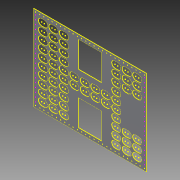
# Autodesk Inventor part: baseplate
Saved by Autodesk Inventor 2014 SP1 (Build 180222100, 222)
## iProperties
Created: 2014-01-05
Part Number: baseplate
Material: Aluminum 6061
Document SubType Name: Sheet Metal
Designer: Arpan
Density: 2.71 g/cm^3
Sheet Metal Rule: Default
Appearance: Aluminum - Flat
Mass: 756.352 g
Surface Area: 3765.33 cm^2
Volume: 279.097 cm^3
Author: Arpan
Autodesk Inventor part; units mm, degrees
ref_plane "YZ Plane" through (0, 0, 0) normal (1, 0, 0) x (0, 1, 0)
ref_plane "XZ Plane" through (0, 0, 0) normal (0, 1, 0) x (-1, 0, 0)
ref_plane "XY Plane" through (0, 0, 0) normal (0, 0, 1) x (1, 0, 0)
sketch "Sketch1" plane through (0, 0, 0) normal (0, 0, 1) x (1, 0, 0)
  line L0 (0, 0) -> (-685.8, 0)
  line L1 (-685.8, 0) -> (-685.8, 516.255)
  line L2 (-685.8, 516.255) -> (0, 516.255)
  line L3 (0, 516.255) -> (0, 0)
  dimension "d0" = 685.8
  dimension "d1" = 516.255
  measures "d0" distance of L1.end L2.end
  measures "d1" distance of L2.end L0.start
extrude "Plate1" add sketch "Sketch1" along normal blind 1.5875
sketch "Sketch4" plane through (0, 0, 1.5875) normal (0, 0, 1) x (1, 0, 0)
  circle A0 centre (-673.1, 503.555) radius 2.0828 projected
  circle A1 centre (-673.1, 12.7) radius 2.0828 projected
extrude "Cut3" cut sketch "Sketch4" against normal blind 1.5875
pattern_linear "Rectangular Pattern2" count 27 spacing 25.4 along (1, 0, 0) of "Cut3"
sketch "Sketch5" plane through (0, 0, 1.5875) normal (0, 0, 1) x (1, 0, 0)
  line L0 (-685.8, 516.255) -> (0, 516.255)
  line L1 (0, 516.255) -> (0, 0)
  line L2 (0, 0) -> (-685.8, 0)
  line L3 (-685.8, 0) -> (-685.8, 516.255)
  line L4 (-25.4, 490.855) -> (-660.4, 490.855)
  line L5 (-660.4, 490.855) -> (-660.4, 25.4)
  line L6 (-660.4, 25.4) -> (-25.4, 25.4)
  line L7 (-25.4, 25.4) -> (-25.4, 490.855)
  line L8 (-660.4, 490.855) -> (-596.9, 490.855)
  line L9 (-596.9, 490.855) -> (-596.9, 444.3095)
  line L10 (-596.9, 444.3095) -> (-660.4, 444.3095)
  line L11 (-660.4, 467.5822) -> (-596.9, 467.5822) construction
  line L12 (-637.1273, 444.3095) -> (-620.1728, 444.3095)
  line L13 (-620.1728, 490.855) -> (-637.1273, 490.855)
  arc A0 (-637.1273, 490.855) -> (-637.1273, 444.3095) centre (-637.1273, 467.5822) ccw
  arc A1 (-620.1728, 444.3095) -> (-620.1728, 490.855) centre (-620.1728, 467.5822) ccw
  line L14 (-620.1728, 487.68) -> (-637.1273, 487.68)
  arc A2 (-637.1273, 487.68) -> (-637.1273, 447.4845) centre (-637.1273, 467.5822) ccw
  line L15 (-637.1273, 447.4845) -> (-620.1728, 447.4845)
  arc A3 (-620.1728, 447.4845) -> (-620.1728, 487.68) centre (-620.1728, 467.5822) ccw
  point P0 (-412.75, 516.255)
  point P1 (-412.75, 0)
  point P2 (-273.05, 0)
  point P3 (-273.05, 516.255)
  point P4 (-628.65, 467.5822)
  dimension "d22" = 25.4
  dimension "d25" = 46.5455
  dimension "d28" = 3.175
  constraints: 34 end point, 10 point on circle, 6 parallel, 5 point on line, 4 centre point, 4 perpendicular, 4 tangent, 2 midpoint, 1 horizontal, 6 other
  measures "d22" distance between parallel lines of L0 L4
  measures "d25" distance of L8.end L9.end
  measures "d28" distance between parallel lines of L8 L14
extrude "Cut5" cut sketch "Sketch5" against normal blind 1.5875 contours A3 L15 A2 L14
pattern_linear "Rectangular Pattern3" count 10 spacing 46.5455 along (0, -1, 0) count 10 spacing 63.5 along (1, 0, 0) of "Cut5"
sketch "Sketch7" plane through (0, 0, 0) normal (0, 0, -1) x (-1, 0, 0)
  line L0 (256.1273, 75.1205) -> (239.1728, 75.1205)
  line L1 (402.7899, 184.15) -> (410.0101, 184.15)
  arc A0 (446.6273, 168.2115) -> (446.6273, 208.407) centre (446.6273, 188.3092) ccw
  arc A1 (429.6728, 208.407) -> (429.6728, 168.2115) centre (429.6728, 188.3092) ccw
  line L2 (412.75, 177.4677) -> (412.75, 152.6053)
  line L3 (273.05, 338.7873) -> (273.05, 363.6497)
  line L4 (283.0101, 332.105) -> (275.7899, 332.105)
  arc A2 (256.1273, 307.848) -> (256.1273, 348.0435) centre (256.1273, 327.9457) ccw
  arc A3 (239.1728, 348.0435) -> (239.1728, 307.848) centre (239.1728, 327.9457) ccw
  line L5 (429.6728, 188.3092) -> (446.6273, 188.3092) construction
  line L6 (429.6728, 168.2115) -> (446.6273, 168.2115)
  line L7 (446.6273, 208.407) -> (429.6728, 208.407)
  arc A4 (429.6728, 208.407) -> (429.6728, 168.2115) centre (429.6728, 188.3092) ccw
  arc A5 (446.6273, 168.2115) -> (446.6273, 208.407) centre (446.6273, 188.3092) ccw
  line L8 (366.1728, 168.2115) -> (383.1273, 168.2115)
  line L9 (383.1273, 208.407) -> (366.1728, 208.407)
  arc A6 (366.1728, 208.407) -> (366.1728, 168.2115) centre (366.1728, 188.3092) ccw
  arc A7 (383.1273, 168.2115) -> (383.1273, 208.407) centre (383.1273, 188.3092) ccw
  line L10 (302.6728, 168.2115) -> (319.6273, 168.2115)
  line L11 (319.6273, 208.407) -> (302.6728, 208.407)
  arc A8 (302.6728, 208.407) -> (302.6728, 168.2115) centre (302.6728, 188.3092) ccw
  arc A9 (319.6273, 168.2115) -> (319.6273, 208.407) centre (319.6273, 188.3092) ccw
  line L12 (239.1728, 168.2115) -> (256.1273, 168.2115)
  line L13 (256.1273, 208.407) -> (239.1728, 208.407)
  arc A10 (239.1728, 208.407) -> (239.1728, 168.2115) centre (239.1728, 188.3092) ccw
  arc A11 (256.1273, 168.2115) -> (256.1273, 208.407) centre (256.1273, 188.3092) ccw
  line L14 (429.6728, 121.666) -> (446.6273, 121.666)
  line L15 (446.6273, 161.8615) -> (429.6728, 161.8615)
  arc A12 (429.6728, 161.8615) -> (429.6728, 121.666) centre (429.6728, 141.7637) ccw
  arc A13 (446.6273, 121.666) -> (446.6273, 161.8615) centre (446.6273, 141.7637) ccw
  line L16 (366.1728, 121.666) -> (383.1273, 121.666)
  line L17 (383.1273, 161.8615) -> (366.1728, 161.8615)
  arc A14 (366.1728, 161.8615) -> (366.1728, 121.666) centre (366.1728, 141.7637) ccw
  arc A15 (383.1273, 121.666) -> (383.1273, 161.8615) centre (383.1273, 141.7637) ccw
  line L18 (302.6728, 121.666) -> (319.6273, 121.666)
  line L19 (319.6273, 161.8615) -> (302.6728, 161.8615)
  arc A16 (302.6728, 161.8615) -> (302.6728, 121.666) centre (302.6728, 141.7637) ccw
  arc A17 (319.6273, 121.666) -> (319.6273, 161.8615) centre (319.6273, 141.7637) ccw
  line L20 (239.1728, 121.666) -> (256.1273, 121.666)
  line L21 (256.1273, 161.8615) -> (239.1728, 161.8615)
  arc A18 (239.1728, 161.8615) -> (239.1728, 121.666) centre (239.1728, 141.7637) ccw
  arc A19 (256.1273, 121.666) -> (256.1273, 161.8615) centre (256.1273, 141.7637) ccw
  line L22 (429.6728, 75.1205) -> (446.6273, 75.1205)
  line L23 (446.6273, 115.316) -> (429.6728, 115.316)
  arc A20 (429.6728, 115.316) -> (429.6728, 75.1205) centre (429.6728, 95.2182) ccw
  arc A21 (446.6273, 75.1205) -> (446.6273, 115.316) centre (446.6273, 95.2182) ccw
  line L24 (366.1728, 75.1205) -> (383.1273, 75.1205)
  line L25 (383.1273, 115.316) -> (366.1728, 115.316)
  arc A22 (366.1728, 115.316) -> (366.1728, 75.1205) centre (366.1728, 95.2182) ccw
  arc A23 (383.1273, 75.1205) -> (383.1273, 115.316) centre (383.1273, 95.2182) ccw
  line L26 (302.6728, 75.1205) -> (319.6273, 75.1205)
  line L27 (319.6273, 115.316) -> (302.6728, 115.316)
  arc A24 (302.6728, 115.316) -> (302.6728, 75.1205) centre (302.6728, 95.2182) ccw
  arc A25 (319.6273, 75.1205) -> (319.6273, 115.316) centre (319.6273, 95.2182) ccw
  line L28 (239.1728, 75.1205) -> (256.1273, 75.1205)
  line L29 (256.1273, 115.316) -> (239.1728, 115.316)
  arc A26 (239.1728, 115.316) -> (239.1728, 75.1205) centre (239.1728, 95.2182) ccw
  arc A27 (256.1273, 75.1205) -> (256.1273, 115.316) centre (256.1273, 95.2182) ccw
  line L30 (429.6728, 28.575) -> (446.6273, 28.575)
  line L31 (446.6273, 68.7705) -> (429.6728, 68.7705)
  arc A28 (429.6728, 68.7705) -> (429.6728, 28.575) centre (429.6728, 48.6727) ccw
  arc A29 (446.6273, 28.575) -> (446.6273, 68.7705) centre (446.6273, 48.6727) ccw
  line L32 (366.1728, 28.575) -> (383.1273, 28.575)
  line L33 (383.1273, 68.7705) -> (366.1728, 68.7705)
  arc A30 (366.1728, 68.7705) -> (366.1728, 28.575) centre (366.1728, 48.6727) ccw
  arc A31 (383.1273, 28.575) -> (383.1273, 68.7705) centre (383.1273, 48.6727) ccw
  line L34 (302.6728, 28.575) -> (319.6273, 28.575)
  line L35 (319.6273, 68.7705) -> (302.6728, 68.7705)
  arc A32 (302.6728, 68.7705) -> (302.6728, 28.575) centre (302.6728, 48.6727) ccw
  arc A33 (319.6273, 28.575) -> (319.6273, 68.7705) centre (319.6273, 48.6727) ccw
  line L36 (239.1728, 28.575) -> (256.1273, 28.575)
  line L37 (256.1273, 68.7705) -> (239.1728, 68.7705)
  arc A34 (239.1728, 68.7705) -> (239.1728, 28.575) centre (239.1728, 48.6727) ccw
  arc A35 (256.1273, 28.575) -> (256.1273, 68.7705) centre (256.1273, 48.6727) ccw
  line L38 (239.1728, 327.9457) -> (256.1273, 327.9457) construction
  line L39 (239.1728, 307.848) -> (256.1273, 307.848)
  line L40 (256.1273, 348.0435) -> (239.1728, 348.0435)
  arc A36 (239.1728, 348.0435) -> (239.1728, 307.848) centre (239.1728, 327.9457) ccw
  arc A37 (256.1273, 307.848) -> (256.1273, 348.0435) centre (256.1273, 327.9457) ccw
  line L41 (239.1728, 354.3935) -> (256.1273, 354.3935)
  line L42 (256.1273, 394.589) -> (239.1728, 394.589)
  arc A38 (239.1728, 394.589) -> (239.1728, 354.3935) centre (239.1728, 374.4912) ccw
  arc A39 (256.1273, 354.3935) -> (256.1273, 394.589) centre (256.1273, 374.4912) ccw
  line L43 (239.1728, 400.939) -> (256.1273, 400.939)
  line L44 (256.1273, 441.1345) -> (239.1728, 441.1345)
  arc A40 (239.1728, 441.1345) -> (239.1728, 400.939) centre (239.1728, 421.0367) ccw
  arc A41 (256.1273, 400.939) -> (256.1273, 441.1345) centre (256.1273, 421.0367) ccw
  line L45 (239.1728, 447.4845) -> (256.1273, 447.4845)
  line L46 (256.1273, 487.68) -> (239.1728, 487.68)
  arc A42 (239.1728, 487.68) -> (239.1728, 447.4845) centre (239.1728, 467.5822) ccw
  arc A43 (256.1273, 447.4845) -> (256.1273, 487.68) centre (256.1273, 467.5822) ccw
  line L47 (302.6728, 307.848) -> (319.6273, 307.848)
  line L48 (319.6273, 348.0435) -> (302.6728, 348.0435)
  arc A44 (302.6728, 348.0435) -> (302.6728, 307.848) centre (302.6728, 327.9457) ccw
  arc A45 (319.6273, 307.848) -> (319.6273, 348.0435) centre (319.6273, 327.9457) ccw
  line L49 (302.6728, 354.3935) -> (319.6273, 354.3935)
  line L50 (319.6273, 394.589) -> (302.6728, 394.589)
  arc A46 (302.6728, 394.589) -> (302.6728, 354.3935) centre (302.6728, 374.4912) ccw
  arc A47 (319.6273, 354.3935) -> (319.6273, 394.589) centre (319.6273, 374.4912) ccw
  line L51 (302.6728, 400.939) -> (319.6273, 400.939)
  line L52 (319.6273, 441.1345) -> (302.6728, 441.1345)
  arc A48 (302.6728, 441.1345) -> (302.6728, 400.939) centre (302.6728, 421.0367) ccw
  arc A49 (319.6273, 400.939) -> (319.6273, 441.1345) centre (319.6273, 421.0367) ccw
  line L53 (302.6728, 447.4845) -> (319.6273, 447.4845)
  line L54 (319.6273, 487.68) -> (302.6728, 487.68)
  arc A50 (302.6728, 487.68) -> (302.6728, 447.4845) centre (302.6728, 467.5822) ccw
  arc A51 (319.6273, 447.4845) -> (319.6273, 487.68) centre (319.6273, 467.5822) ccw
  line L55 (366.1728, 307.848) -> (383.1273, 307.848)
  line L56 (383.1273, 348.0435) -> (366.1728, 348.0435)
  arc A52 (366.1728, 348.0435) -> (366.1728, 307.848) centre (366.1728, 327.9457) ccw
  arc A53 (383.1273, 307.848) -> (383.1273, 348.0435) centre (383.1273, 327.9457) ccw
  line L57 (366.1728, 354.3935) -> (383.1273, 354.3935)
  line L58 (383.1273, 394.589) -> (366.1728, 394.589)
  arc A54 (366.1728, 394.589) -> (366.1728, 354.3935) centre (366.1728, 374.4912) ccw
  arc A55 (383.1273, 354.3935) -> (383.1273, 394.589) centre (383.1273, 374.4912) ccw
  line L59 (366.1728, 400.939) -> (383.1273, 400.939)
  line L60 (383.1273, 441.1345) -> (366.1728, 441.1345)
  arc A56 (366.1728, 441.1345) -> (366.1728, 400.939) centre (366.1728, 421.0367) ccw
  arc A57 (383.1273, 400.939) -> (383.1273, 441.1345) centre (383.1273, 421.0367) ccw
  line L61 (366.1728, 447.4845) -> (383.1273, 447.4845)
  line L62 (383.1273, 487.68) -> (366.1728, 487.68)
  arc A58 (366.1728, 487.68) -> (366.1728, 447.4845) centre (366.1728, 467.5822) ccw
  arc A59 (383.1273, 447.4845) -> (383.1273, 487.68) centre (383.1273, 467.5822) ccw
  line L63 (429.6728, 307.848) -> (446.6273, 307.848)
  line L64 (446.6273, 348.0435) -> (429.6728, 348.0435)
  arc A60 (429.6728, 348.0435) -> (429.6728, 307.848) centre (429.6728, 327.9457) ccw
  arc A61 (446.6273, 307.848) -> (446.6273, 348.0435) centre (446.6273, 327.9457) ccw
  line L65 (429.6728, 354.3935) -> (446.6273, 354.3935)
  line L66 (446.6273, 394.589) -> (429.6728, 394.589)
  arc A62 (429.6728, 394.589) -> (429.6728, 354.3935) centre (429.6728, 374.4912) ccw
  arc A63 (446.6273, 354.3935) -> (446.6273, 394.589) centre (446.6273, 374.4912) ccw
  line L67 (429.6728, 400.939) -> (446.6273, 400.939)
  line L68 (446.6273, 441.1345) -> (429.6728, 441.1345)
  arc A64 (429.6728, 441.1345) -> (429.6728, 400.939) centre (429.6728, 421.0367) ccw
  arc A65 (446.6273, 400.939) -> (446.6273, 441.1345) centre (446.6273, 421.0367) ccw
  line L69 (429.6728, 447.4845) -> (446.6273, 447.4845)
  line L70 (446.6273, 487.68) -> (429.6728, 487.68)
  arc A66 (429.6728, 487.68) -> (429.6728, 447.4845) centre (429.6728, 467.5822) ccw
  arc A67 (446.6273, 447.4845) -> (446.6273, 487.68) centre (446.6273, 467.5822) ccw
  point P0 (438.15, 188.3092)
  point P1 (247.65, 327.9457)
  dimension "d46" = 63.5
  dimension "d49" = 46.5455
  dimension "d54" = 46.5455
  dimension "d57" = 63.5
  measures "d46" distance of L6.start L8.start
  measures "d49" distance of L6.start L14.start
  measures "d54" distance of L40.start L42.start
  measures "d57" distance of L40.start L48.start
sheet face with bend "Face2" sketch "Sketch7" thickness 1.5875 toward (0, 0, 1) bend radius 1.5875 relief tear relief width 1.5875 relief depth 0.7937
bend "Bend1"
sketch "Sketch2" plane through (0, 0, 1.5875) normal (0, 0, 1) x (1, 0, 0)
  line L0 (0, 0) -> (-685.8, 0) projected
  line L1 (-685.8, 516.255) -> (0, 516.255) projected
  line L2 (-342.9, 516.255) -> (-412.75, 516.255)
  line L3 (-412.75, 516.255) -> (-412.75, 332.105)
  line L4 (-412.75, 332.105) -> (-273.05, 332.105)
  line L5 (-273.05, 332.105) -> (-273.05, 516.255)
  line L6 (-412.75, 0) -> (-412.75, 184.15)
  line L7 (-412.75, 184.15) -> (-273.05, 184.15)
  line L8 (-273.05, 184.15) -> (-273.05, 0)
  line L9 (-412.75, 0) -> (-412.75, 25.4)
  line L10 (-412.75, 25.4) -> (-273.05, 25.4)
  line L11 (-273.05, 516.255) -> (-273.05, 490.855)
  line L12 (-273.05, 490.855) -> (-412.75, 490.855)
  dimension "d3" = 69.85
  dimension "d4" = 184.15
  dimension "d5" = 139.7
  dimension "d6" = 184.15
  dimension "d23" = 25.4
  dimension "d24" = 25.4
  constraints: 22 end point, 8 point on line, 6 perpendicular, 2 parallel, 1 midpoint
  measures "d3" distance of L2.start L2.end
  measures "d4" distance of L2.end L3.end
  measures "d5" distance of L3.end L4.end
  measures "d6" distance of L6.start L6.end
  measures "d23" distance of L6.start L9.end
  measures "d24" distance of L5.end L11.end
extrude "Cut6" cut sketch "Sketch2" against normal blind 1.5875 contours L10 L6 L7 L8 | L12 L5 L4 L3
sketch "Sketch8" plane through (0, 0, 0) normal (0, 0, -1) x (-1, 0, 0)
  line L0 (273.05, 490.855) -> (412.75, 490.855)
  arc A0 (65.6273, 168.2115) -> (65.6273, 208.407) centre (65.6273, 188.3092) ccw
  line L1 (65.6273, 168.2115) -> (48.6728, 168.2115)
  arc A1 (48.6728, 208.407) -> (48.6728, 168.2115) centre (48.6728, 188.3092) ccw
  line L2 (48.6728, 208.407) -> (65.6273, 208.407)
  line L3 (48.6728, 188.3092) -> (65.6273, 188.3092) construction
  line L4 (48.6728, 168.2115) -> (65.6273, 168.2115)
  line L5 (65.6273, 208.407) -> (48.6728, 208.407)
  arc A2 (48.6728, 208.407) -> (48.6728, 168.2115) centre (48.6728, 188.3092) ccw
  arc A3 (65.6273, 168.2115) -> (65.6273, 208.407) centre (65.6273, 188.3092) ccw
  point P0 (57.15, 188.3092)
sheet face with bend "Face3" sketch "Sketch8" thickness 1.5875 toward (0, 0, 1) bend radius 1.5875 relief tear relief width 1.5875 relief depth 0.7937
bend "Bend2"
pattern_linear "Rectangular Pattern4" count 2 spacing 63.5 along (-1, 0, 0) count 4 spacing 46.5455 along (0, 1, 0) of "Face3"
sketch "Sketch9" plane through (0, 0, 0) normal (0, 0, -1) x (-1, 0, 0)
  line L0 (273.05, 332.105) -> (273.05, 490.855) projected
  line L1 (273.05, 490.855) -> (412.75, 490.855) projected
  line L2 (412.75, 490.855) -> (412.75, 332.105) projected
  line L3 (412.75, 332.105) -> (273.05, 332.105) projected
  line L4 (412.75, 25.4) -> (273.05, 25.4) projected
  line L5 (273.05, 25.4) -> (273.05, 184.15) projected
  line L6 (273.05, 184.15) -> (412.75, 184.15) projected
  line L7 (412.75, 184.15) -> (412.75, 25.4) projected
  arc A0 (65.6272, 28.575) -> (65.6272, 68.7705) centre (65.6272, 48.6727) ccw projected
  line L8 (65.6272, 28.575) -> (48.6728, 28.575) projected
  arc A1 (48.6728, 68.7705) -> (48.6728, 28.575) centre (48.6728, 48.6727) ccw projected
  line L9 (48.6728, 68.7705) -> (65.6272, 68.7705) projected
  arc A2 (65.6273, 75.1205) -> (65.6273, 115.316) centre (65.6273, 95.2182) ccw projected
  line L10 (65.6273, 75.1205) -> (48.6728, 75.1205) projected
  arc A3 (48.6728, 115.316) -> (48.6728, 75.1205) centre (48.6728, 95.2182) ccw projected
  line L11 (48.6728, 115.316) -> (65.6273, 115.316) projected
  arc A4 (65.6273, 121.666) -> (65.6273, 161.8615) centre (65.6273, 141.7637) ccw projected
  line L12 (65.6273, 121.666) -> (48.6728, 121.666) projected
  arc A5 (48.6728, 161.8615) -> (48.6728, 121.666) centre (48.6728, 141.7637) ccw projected
  line L13 (48.6728, 161.8615) -> (65.6273, 161.8615) projected
  arc A6 (65.6273, 354.3935) -> (65.6273, 394.589) centre (65.6273, 374.4912) ccw projected
  line L14 (65.6273, 354.3935) -> (48.6728, 354.3935) projected
  arc A7 (48.6728, 394.589) -> (48.6728, 354.3935) centre (48.6728, 374.4912) ccw projected
  line L15 (48.6728, 394.589) -> (65.6273, 394.589) projected
  arc A8 (65.6273, 400.939) -> (65.6273, 441.1345) centre (65.6273, 421.0367) ccw projected
  line L16 (65.6273, 400.939) -> (48.6728, 400.939) projected
  arc A9 (48.6728, 441.1345) -> (48.6728, 400.939) centre (48.6728, 421.0367) ccw projected
  line L17 (48.6728, 441.1345) -> (65.6273, 441.1345) projected
  arc A10 (65.6273, 447.4845) -> (65.6273, 487.68) centre (65.6273, 467.5822) ccw projected
  line L18 (65.6273, 447.4845) -> (48.6728, 447.4845) projected
  arc A11 (48.6728, 487.68) -> (48.6728, 447.4845) centre (48.6728, 467.5822) ccw projected
  line L19 (48.6728, 487.68) -> (65.6273, 487.68) projected
  arc A12 (129.1272, 28.575) -> (129.1272, 68.7705) centre (129.1272, 48.6727) ccw projected
  line L20 (129.1272, 28.575) -> (112.1728, 28.575) projected
  arc A13 (112.1728, 68.7705) -> (112.1728, 28.575) centre (112.1728, 48.6727) ccw projected
  line L21 (112.1728, 68.7705) -> (129.1272, 68.7705) projected
  arc A14 (129.1273, 75.1205) -> (129.1273, 115.316) centre (129.1273, 95.2182) ccw projected
  line L22 (129.1273, 75.1205) -> (112.1728, 75.1205) projected
  arc A15 (112.1728, 115.316) -> (112.1728, 75.1205) centre (112.1728, 95.2182) ccw projected
  line L23 (112.1728, 115.316) -> (129.1273, 115.316) projected
  arc A16 (129.1273, 121.666) -> (129.1273, 161.8615) centre (129.1273, 141.7637) ccw projected
  line L24 (129.1273, 121.666) -> (112.1728, 121.666) projected
  arc A17 (112.1728, 161.8615) -> (112.1728, 121.666) centre (112.1728, 141.7637) ccw projected
  line L25 (112.1728, 161.8615) -> (129.1273, 161.8615) projected
  arc A18 (129.1273, 354.3935) -> (129.1273, 394.589) centre (129.1273, 374.4912) ccw projected
  line L26 (129.1273, 354.3935) -> (112.1728, 354.3935) projected
  arc A19 (112.1728, 394.589) -> (112.1728, 354.3935) centre (112.1728, 374.4912) ccw projected
  line L27 (112.1728, 394.589) -> (129.1273, 394.589) projected
  arc A20 (129.1273, 400.939) -> (129.1273, 441.1345) centre (129.1273, 421.0367) ccw projected
  line L28 (129.1273, 400.939) -> (112.1728, 400.939) projected
  arc A21 (112.1728, 441.1345) -> (112.1728, 400.939) centre (112.1728, 421.0367) ccw projected
  line L29 (112.1728, 441.1345) -> (129.1273, 441.1345) projected
  arc A22 (129.1273, 447.4845) -> (129.1273, 487.68) centre (129.1273, 467.5822) ccw projected
  line L30 (129.1273, 447.4845) -> (112.1728, 447.4845) projected
  arc A23 (112.1728, 487.68) -> (112.1728, 447.4845) centre (112.1728, 467.5822) ccw projected
  line L31 (112.1728, 487.68) -> (129.1273, 487.68) projected
  arc A24 (192.6272, 28.575) -> (192.6272, 68.7705) centre (192.6272, 48.6727) ccw projected
  line L32 (192.6272, 28.575) -> (175.6728, 28.575) projected
  arc A25 (175.6728, 68.7705) -> (175.6728, 28.575) centre (175.6728, 48.6727) ccw projected
  line L33 (175.6728, 68.7705) -> (192.6272, 68.7705) projected
  arc A26 (192.6273, 75.1205) -> (192.6273, 115.316) centre (192.6273, 95.2182) ccw projected
  line L34 (192.6273, 75.1205) -> (175.6728, 75.1205) projected
  arc A27 (175.6728, 115.316) -> (175.6728, 75.1205) centre (175.6728, 95.2182) ccw projected
  line L35 (175.6728, 115.316) -> (192.6273, 115.316) projected
  arc A28 (192.6273, 121.666) -> (192.6273, 161.8615) centre (192.6273, 141.7637) ccw projected
  line L36 (192.6273, 121.666) -> (175.6728, 121.666) projected
  arc A29 (175.6728, 161.8615) -> (175.6728, 121.666) centre (175.6728, 141.7637) ccw projected
  line L37 (175.6728, 161.8615) -> (192.6273, 161.8615) projected
  arc A30 (192.6273, 168.2115) -> (192.6273, 208.407) centre (192.6273, 188.3092) ccw projected
  line L38 (192.6273, 168.2115) -> (175.6728, 168.2115) projected
  arc A31 (175.6728, 208.407) -> (175.6728, 168.2115) centre (175.6728, 188.3092) ccw projected
  line L39 (175.6728, 208.407) -> (192.6273, 208.407) projected
  arc A32 (192.6273, 214.757) -> (192.6273, 254.9525) centre (192.6273, 234.8547) ccw projected
  line L40 (192.6273, 214.757) -> (175.6728, 214.757) projected
  arc A33 (175.6728, 254.9525) -> (175.6728, 214.757) centre (175.6728, 234.8547) ccw projected
  line L41 (175.6728, 254.9525) -> (192.6273, 254.9525) projected
  arc A34 (192.6273, 261.3025) -> (192.6273, 301.498) centre (192.6273, 281.4002) ccw projected
  line L42 (192.6273, 261.3025) -> (175.6728, 261.3025) projected
  arc A35 (175.6728, 301.498) -> (175.6728, 261.3025) centre (175.6728, 281.4002) ccw projected
  line L43 (175.6728, 301.498) -> (192.6273, 301.498) projected
  arc A36 (192.6273, 307.848) -> (192.6273, 348.0435) centre (192.6273, 327.9457) ccw projected
  line L44 (192.6273, 307.848) -> (175.6728, 307.848) projected
  arc A37 (175.6728, 348.0435) -> (175.6728, 307.848) centre (175.6728, 327.9457) ccw projected
  line L45 (175.6728, 348.0435) -> (192.6273, 348.0435) projected
  arc A38 (192.6273, 354.3935) -> (192.6273, 394.589) centre (192.6273, 374.4912) ccw projected
  line L46 (192.6273, 354.3935) -> (175.6728, 354.3935) projected
  arc A39 (175.6728, 394.589) -> (175.6728, 354.3935) centre (175.6728, 374.4912) ccw projected
  line L47 (175.6728, 394.589) -> (192.6273, 394.589) projected
  arc A40 (192.6273, 400.939) -> (192.6273, 441.1345) centre (192.6273, 421.0367) ccw projected
  line L48 (192.6273, 400.939) -> (175.6728, 400.939) projected
  arc A41 (175.6728, 441.1345) -> (175.6728, 400.939) centre (175.6728, 421.0367) ccw projected
  line L49 (175.6728, 441.1345) -> (192.6273, 441.1345) projected
  arc A42 (192.6273, 447.4845) -> (192.6273, 487.68) centre (192.6273, 467.5822) ccw projected
  line L50 (192.6273, 447.4845) -> (175.6728, 447.4845) projected
  arc A43 (175.6728, 487.68) -> (175.6728, 447.4845) centre (175.6728, 467.5822) ccw projected
  line L51 (175.6728, 487.68) -> (192.6273, 487.68) projected
  arc A44 (256.1273, 214.757) -> (256.1273, 254.9525) centre (256.1273, 234.8547) ccw projected
  line L52 (256.1273, 214.757) -> (239.1728, 214.757) projected
  arc A45 (239.1728, 254.9525) -> (239.1728, 214.757) centre (239.1728, 234.8547) ccw projected
  line L53 (239.1728, 254.9525) -> (256.1273, 254.9525) projected
  arc A46 (256.1273, 261.3025) -> (256.1273, 301.498) centre (256.1273, 281.4002) ccw projected
  line L54 (256.1273, 261.3025) -> (239.1728, 261.3025) projected
  arc A47 (239.1728, 301.498) -> (239.1728, 261.3025) centre (239.1728, 281.4002) ccw projected
  line L55 (239.1728, 301.498) -> (256.1273, 301.498) projected
  arc A48 (319.6273, 214.757) -> (319.6273, 254.9525) centre (319.6273, 234.8547) ccw projected
  line L56 (319.6273, 214.757) -> (302.6728, 214.757) projected
  arc A49 (302.6728, 254.9525) -> (302.6728, 214.757) centre (302.6728, 234.8547) ccw projected
  line L57 (302.6728, 254.9525) -> (319.6273, 254.9525) projected
  arc A50 (319.6273, 261.3025) -> (319.6273, 301.498) centre (319.6273, 281.4002) ccw projected
  line L58 (319.6273, 261.3025) -> (302.6728, 261.3025) projected
  arc A51 (302.6728, 301.498) -> (302.6728, 261.3025) centre (302.6728, 281.4002) ccw projected
  line L59 (302.6728, 301.498) -> (319.6273, 301.498) projected
  arc A52 (383.1273, 214.757) -> (383.1273, 254.9525) centre (383.1273, 234.8547) ccw projected
  line L60 (383.1273, 214.757) -> (366.1728, 214.757) projected
  arc A53 (366.1728, 254.9525) -> (366.1728, 214.757) centre (366.1728, 234.8547) ccw projected
  line L61 (366.1728, 254.9525) -> (383.1273, 254.9525) projected
  arc A54 (383.1273, 261.3025) -> (383.1273, 301.498) centre (383.1273, 281.4002) ccw projected
  line L62 (383.1273, 261.3025) -> (366.1728, 261.3025) projected
  arc A55 (366.1728, 301.498) -> (366.1728, 261.3025) centre (366.1728, 281.4002) ccw projected
  line L63 (366.1728, 301.498) -> (383.1273, 301.498) projected
  arc A56 (446.6273, 214.757) -> (446.6273, 254.9525) centre (446.6273, 234.8547) ccw projected
  line L64 (446.6273, 214.757) -> (429.6728, 214.757) projected
  arc A57 (429.6728, 254.9525) -> (429.6728, 214.757) centre (429.6728, 234.8547) ccw projected
  line L65 (429.6728, 254.9525) -> (446.6273, 254.9525) projected
  arc A58 (446.6273, 261.3025) -> (446.6273, 301.498) centre (446.6273, 281.4002) ccw projected
  line L66 (446.6273, 261.3025) -> (429.6728, 261.3025) projected
  arc A59 (429.6728, 301.498) -> (429.6728, 261.3025) centre (429.6728, 281.4002) ccw projected
  line L67 (429.6728, 301.498) -> (446.6273, 301.498) projected
  arc A60 (510.1272, 28.575) -> (510.1272, 68.7705) centre (510.1272, 48.6727) ccw projected
  line L68 (510.1272, 28.575) -> (493.1728, 28.575) projected
  arc A61 (493.1728, 68.7705) -> (493.1728, 28.575) centre (493.1728, 48.6727) ccw projected
  line L69 (493.1728, 68.7705) -> (510.1272, 68.7705) projected
  arc A62 (510.1272, 75.1205) -> (510.1272, 115.316) centre (510.1272, 95.2182) ccw projected
  line L70 (510.1272, 75.1205) -> (493.1728, 75.1205) projected
  arc A63 (493.1728, 115.316) -> (493.1728, 75.1205) centre (493.1728, 95.2182) ccw projected
  line L71 (493.1728, 115.316) -> (510.1272, 115.316) projected
  arc A64 (510.1272, 121.666) -> (510.1272, 161.8615) centre (510.1272, 141.7637) ccw projected
  line L72 (510.1272, 121.666) -> (493.1728, 121.666) projected
  arc A65 (493.1728, 161.8615) -> (493.1728, 121.666) centre (493.1728, 141.7637) ccw projected
  line L73 (493.1728, 161.8615) -> (510.1272, 161.8615) projected
  arc A66 (510.1273, 168.2115) -> (510.1273, 208.407) centre (510.1273, 188.3092) ccw projected
  line L74 (510.1273, 168.2115) -> (493.1728, 168.2115) projected
  arc A67 (493.1728, 208.407) -> (493.1728, 168.2115) centre (493.1728, 188.3092) ccw projected
  line L75 (493.1728, 208.407) -> (510.1273, 208.407) projected
  arc A68 (510.1273, 214.757) -> (510.1273, 254.9525) centre (510.1273, 234.8547) ccw projected
  line L76 (510.1273, 214.757) -> (493.1728, 214.757) projected
  arc A69 (493.1728, 254.9525) -> (493.1728, 214.757) centre (493.1728, 234.8547) ccw projected
  line L77 (493.1728, 254.9525) -> (510.1273, 254.9525) projected
  arc A70 (510.1273, 261.3025) -> (510.1273, 301.498) centre (510.1273, 281.4002) ccw projected
  line L78 (510.1273, 261.3025) -> (493.1728, 261.3025) projected
  arc A71 (493.1728, 301.498) -> (493.1728, 261.3025) centre (493.1728, 281.4002) ccw projected
  line L79 (493.1728, 301.498) -> (510.1273, 301.498) projected
  arc A72 (510.1273, 307.848) -> (510.1273, 348.0435) centre (510.1273, 327.9457) ccw projected
  line L80 (510.1273, 307.848) -> (493.1728, 307.848) projected
  arc A73 (493.1728, 348.0435) -> (493.1728, 307.848) centre (493.1728, 327.9457) ccw projected
  line L81 (493.1728, 348.0435) -> (510.1273, 348.0435) projected
  arc A74 (510.1273, 354.3935) -> (510.1273, 394.589) centre (510.1273, 374.4912) ccw projected
  line L82 (510.1273, 354.3935) -> (493.1728, 354.3935) projected
  arc A75 (493.1728, 394.589) -> (493.1728, 354.3935) centre (493.1728, 374.4912) ccw projected
  line L83 (493.1728, 394.589) -> (510.1273, 394.589) projected
  arc A76 (510.1273, 400.939) -> (510.1273, 441.1345) centre (510.1273, 421.0367) ccw projected
  line L84 (510.1273, 400.939) -> (493.1728, 400.939) projected
  arc A77 (493.1728, 441.1345) -> (493.1728, 400.939) centre (493.1728, 421.0367) ccw projected
  line L85 (493.1728, 441.1345) -> (510.1273, 441.1345) projected
  arc A78 (510.1273, 447.4845) -> (510.1273, 487.68) centre (510.1273, 467.5822) ccw projected
  line L86 (510.1273, 447.4845) -> (493.1728, 447.4845) projected
  arc A79 (493.1728, 487.68) -> (493.1728, 447.4845) centre (493.1728, 467.5822) ccw projected
  line L87 (493.1728, 487.68) -> (510.1273, 487.68) projected
  arc A80 (573.6273, 28.575) -> (573.6273, 68.7705) centre (573.6273, 48.6727) ccw projected
  line L88 (573.6273, 28.575) -> (556.6728, 28.575) projected
  arc A81 (556.6728, 68.7705) -> (556.6728, 28.575) centre (556.6728, 48.6727) ccw projected
  line L89 (556.6728, 68.7705) -> (573.6273, 68.7705) projected
  arc A82 (573.6273, 75.1205) -> (573.6273, 115.316) centre (573.6273, 95.2182) ccw projected
  line L90 (573.6273, 75.1205) -> (556.6728, 75.1205) projected
  arc A83 (556.6728, 115.316) -> (556.6728, 75.1205) centre (556.6728, 95.2182) ccw projected
  line L91 (556.6728, 115.316) -> (573.6273, 115.316) projected
  arc A84 (573.6273, 121.666) -> (573.6273, 161.8615) centre (573.6273, 141.7637) ccw projected
  line L92 (573.6273, 121.666) -> (556.6728, 121.666) projected
  arc A85 (556.6728, 161.8615) -> (556.6728, 121.666) centre (556.6728, 141.7637) ccw projected
  line L93 (556.6728, 161.8615) -> (573.6273, 161.8615) projected
  arc A86 (573.6273, 168.2115) -> (573.6273, 208.407) centre (573.6273, 188.3092) ccw projected
  line L94 (573.6273, 168.2115) -> (556.6728, 168.2115) projected
  arc A87 (556.6728, 208.407) -> (556.6728, 168.2115) centre (556.6728, 188.3092) ccw projected
  line L95 (556.6728, 208.407) -> (573.6273, 208.407) projected
  arc A88 (573.6273, 214.757) -> (573.6273, 254.9525) centre (573.6273, 234.8547) ccw projected
  line L96 (573.6273, 214.757) -> (556.6728, 214.757) projected
  arc A89 (556.6728, 254.9525) -> (556.6728, 214.757) centre (556.6728, 234.8547) ccw projected
  line L97 (556.6728, 254.9525) -> (573.6273, 254.9525) projected
  arc A90 (573.6273, 261.3025) -> (573.6273, 301.498) centre (573.6273, 281.4002) ccw projected
  line L98 (573.6273, 261.3025) -> (556.6728, 261.3025) projected
  arc A91 (556.6728, 301.498) -> (556.6728, 261.3025) centre (556.6728, 281.4002) ccw projected
  line L99 (556.6728, 301.498) -> (573.6273, 301.498) projected
  arc A92 (573.6273, 307.848) -> (573.6273, 348.0435) centre (573.6273, 327.9457) ccw projected
  line L100 (573.6273, 307.848) -> (556.6728, 307.848) projected
  arc A93 (556.6728, 348.0435) -> (556.6728, 307.848) centre (556.6728, 327.9457) ccw projected
  line L101 (556.6728, 348.0435) -> (573.6273, 348.0435) projected
  arc A94 (573.6273, 354.3935) -> (573.6273, 394.589) centre (573.6273, 374.4912) ccw projected
  line L102 (573.6273, 354.3935) -> (556.6728, 354.3935) projected
  arc A95 (556.6728, 394.589) -> (556.6728, 354.3935) centre (556.6728, 374.4912) ccw projected
  line L103 (556.6728, 394.589) -> (573.6273, 394.589) projected
  arc A96 (573.6273, 400.939) -> (573.6273, 441.1345) centre (573.6273, 421.0367) ccw projected
  line L104 (573.6273, 400.939) -> (556.6728, 400.939) projected
  arc A97 (556.6728, 441.1345) -> (556.6728, 400.939) centre (556.6728, 421.0367) ccw projected
  line L105 (556.6728, 441.1345) -> (573.6273, 441.1345) projected
  arc A98 (573.6273, 447.4845) -> (573.6273, 487.68) centre (573.6273, 467.5822) ccw projected
  line L106 (573.6273, 447.4845) -> (556.6728, 447.4845) projected
  arc A99 (556.6728, 487.68) -> (556.6728, 447.4845) centre (556.6728, 467.5822) ccw projected
  line L107 (556.6728, 487.68) -> (573.6273, 487.68) projected
  arc A100 (637.1272, 28.575) -> (637.1272, 68.7705) centre (637.1272, 48.6727) ccw projected
  line L108 (637.1272, 28.575) -> (620.1728, 28.575) projected
  arc A101 (620.1728, 68.7705) -> (620.1728, 28.575) centre (620.1728, 48.6727) ccw projected
  line L109 (620.1728, 68.7705) -> (637.1272, 68.7705) projected
  arc A102 (637.1273, 75.1205) -> (637.1273, 115.316) centre (637.1273, 95.2182) ccw projected
  line L110 (637.1273, 75.1205) -> (620.1728, 75.1205) projected
  arc A103 (620.1728, 115.316) -> (620.1728, 75.1205) centre (620.1728, 95.2182) ccw projected
  line L111 (620.1728, 115.316) -> (637.1273, 115.316) projected
  arc A104 (637.1273, 121.666) -> (637.1273, 161.8615) centre (637.1273, 141.7637) ccw projected
  line L112 (637.1273, 121.666) -> (620.1728, 121.666) projected
  arc A105 (620.1728, 161.8615) -> (620.1728, 121.666) centre (620.1728, 141.7637) ccw projected
  line L113 (620.1728, 161.8615) -> (637.1273, 161.8615) projected
  arc A106 (637.1273, 168.2115) -> (637.1273, 208.407) centre (637.1273, 188.3092) ccw projected
  line L114 (637.1273, 168.2115) -> (620.1728, 168.2115) projected
  arc A107 (620.1728, 208.407) -> (620.1728, 168.2115) centre (620.1728, 188.3092) ccw projected
  line L115 (620.1728, 208.407) -> (637.1273, 208.407) projected
  arc A108 (637.1273, 214.757) -> (637.1273, 254.9525) centre (637.1273, 234.8547) ccw projected
  line L116 (637.1273, 214.757) -> (620.1728, 214.757) projected
  arc A109 (620.1728, 254.9525) -> (620.1728, 214.757) centre (620.1728, 234.8547) ccw projected
  line L117 (620.1728, 254.9525) -> (637.1273, 254.9525) projected
  arc A110 (637.1273, 261.3025) -> (637.1273, 301.498) centre (637.1273, 281.4002) ccw projected
  line L118 (637.1273, 261.3025) -> (620.1728, 261.3025) projected
  arc A111 (620.1728, 301.498) -> (620.1728, 261.3025) centre (620.1728, 281.4002) ccw projected
  line L119 (620.1728, 301.498) -> (637.1273, 301.498) projected
  arc A112 (637.1273, 307.848) -> (637.1273, 348.0435) centre (637.1273, 327.9457) ccw projected
  line L120 (637.1273, 307.848) -> (620.1728, 307.848) projected
  arc A113 (620.1728, 348.0435) -> (620.1728, 307.848) centre (620.1728, 327.9457) ccw projected
  line L121 (620.1728, 348.0435) -> (637.1273, 348.0435) projected
  arc A114 (637.1273, 354.3935) -> (637.1273, 394.589) centre (637.1273, 374.4912) ccw projected
  line L122 (637.1273, 354.3935) -> (620.1728, 354.3935) projected
  arc A115 (620.1728, 394.589) -> (620.1728, 354.3935) centre (620.1728, 374.4912) ccw projected
  line L123 (620.1728, 394.589) -> (637.1273, 394.589) projected
  arc A116 (637.1273, 400.939) -> (637.1273, 441.1345) centre (637.1273, 421.0367) ccw projected
  line L124 (637.1273, 400.939) -> (620.1728, 400.939) projected
  arc A117 (620.1728, 441.1345) -> (620.1728, 400.939) centre (620.1728, 421.0367) ccw projected
  line L125 (620.1728, 441.1345) -> (637.1273, 441.1345) projected
  arc A118 (637.1273, 447.4845) -> (637.1273, 487.68) centre (637.1273, 467.5822) ccw projected
  line L126 (637.1273, 447.4845) -> (620.1728, 447.4845) projected
  arc A119 (620.1728, 487.68) -> (620.1728, 447.4845) centre (620.1728, 467.5822) ccw projected
  line L127 (620.1728, 487.68) -> (637.1273, 487.68) projected
  circle A120 centre (12.7, 503.555) radius 2.0828 projected
  circle A121 centre (12.7, 12.7) radius 2.0828 projected
  circle A122 centre (38.1, 503.555) radius 2.0828 projected
  circle A123 centre (38.1, 12.7) radius 2.0828 projected
  circle A124 centre (63.5, 503.555) radius 2.0828 projected
  circle A125 centre (63.5, 12.7) radius 2.0828 projected
  circle A126 centre (88.9, 503.555) radius 2.0828 projected
  circle A127 centre (88.9, 12.7) radius 2.0828 projected
  circle A128 centre (114.3, 503.555) radius 2.0828 projected
  circle A129 centre (114.3, 12.7) radius 2.0828 projected
  circle A130 centre (139.7, 503.555) radius 2.0828 projected
  circle A131 centre (139.7, 12.7) radius 2.0828 projected
  circle A132 centre (165.1, 503.555) radius 2.0828 projected
  circle A133 centre (165.1, 12.7) radius 2.0828 projected
  circle A134 centre (190.5, 503.555) radius 2.0828 projected
  circle A135 centre (190.5, 12.7) radius 2.0828 projected
  circle A136 centre (215.9, 503.555) radius 2.0828 projected
  circle A137 centre (215.9, 12.7) radius 2.0828 projected
  circle A138 centre (241.3, 503.555) radius 2.0828 projected
  circle A139 centre (241.3, 12.7) radius 2.0828 projected
  circle A140 centre (266.7, 503.555) radius 2.0828 projected
  circle A141 centre (266.7, 12.7) radius 2.0828 projected
  circle A142 centre (292.1, 503.555) radius 2.0828 projected
  circle A143 centre (292.1, 12.7) radius 2.0828 projected
  circle A144 centre (317.5, 503.555) radius 2.0828 projected
  circle A145 centre (317.5, 12.7) radius 2.0828 projected
  circle A146 centre (342.9, 503.555) radius 2.0828 projected
  circle A147 centre (342.9, 12.7) radius 2.0828 projected
  circle A148 centre (368.3, 503.555) radius 2.0828 projected
  circle A149 centre (368.3, 12.7) radius 2.0828 projected
  circle A150 centre (393.7, 503.555) radius 2.0828 projected
  circle A151 centre (393.7, 12.7) radius 2.0828 projected
  circle A152 centre (419.1, 503.555) radius 2.0828 projected
  circle A153 centre (419.1, 12.7) radius 2.0828 projected
  circle A154 centre (444.5, 503.555) radius 2.0828 projected
  circle A155 centre (444.5, 12.7) radius 2.0828 projected
  circle A156 centre (469.9, 503.555) radius 2.0828 projected
  circle A157 centre (469.9, 12.7) radius 2.0828 projected
  circle A158 centre (495.3, 503.555) radius 2.0828 projected
  circle A159 centre (495.3, 12.7) radius 2.0828 projected
  circle A160 centre (520.7, 503.555) radius 2.0828 projected
  circle A161 centre (520.7, 12.7) radius 2.0828 projected
  circle A162 centre (546.1, 503.555) radius 2.0828 projected
  circle A163 centre (546.1, 12.7) radius 2.0828 projected
  circle A164 centre (571.5, 503.555) radius 2.0828 projected
  circle A165 centre (571.5, 12.7) radius 2.0828 projected
  circle A166 centre (596.9, 503.555) radius 2.0828 projected
  circle A167 centre (596.9, 12.7) radius 2.0828 projected
  circle A168 centre (622.3, 503.555) radius 2.0828 projected
  circle A169 centre (622.3, 12.7) radius 2.0828 projected
  circle A170 centre (647.7, 503.555) radius 2.0828 projected
  circle A171 centre (647.7, 12.7) radius 2.0828 projected
  circle A172 centre (673.1, 503.555) radius 2.0828 projected
  circle A173 centre (673.1, 12.7) radius 2.0828 projected
  circle A174 centre (12.7, 31.115) radius 2.0828 projected
  circle A175 centre (12.7, 56.515) radius 2.0828 projected
  circle A176 centre (12.7, 81.915) radius 2.0828 projected
  circle A177 centre (12.7, 107.315) radius 2.0828 projected
  circle A178 centre (12.7, 132.715) radius 2.0828 projected
  circle A179 centre (12.7, 158.115) radius 2.0828 projected
  circle A180 centre (12.7, 183.515) radius 2.0828 projected
  circle A181 centre (12.7, 208.915) radius 2.0828 projected
  circle A182 centre (12.7, 234.315) radius 2.0828 projected
  circle A183 centre (12.7, 259.715) radius 2.0828 projected
  circle A184 centre (12.7, 285.115) radius 2.0828 projected
  circle A185 centre (12.7, 310.515) radius 2.0828 projected
  circle A186 centre (12.7, 335.915) radius 2.0828 projected
  circle A187 centre (12.7, 361.315) radius 2.0828 projected
  circle A188 centre (12.7, 386.715) radius 2.0828 projected
  circle A189 centre (12.7, 412.115) radius 2.0828 projected
  circle A190 centre (12.7, 437.515) radius 2.0828 projected
  circle A191 centre (12.7, 462.915) radius 2.0828 projected
  circle A192 centre (12.7, 488.315) radius 2.0828 projected
  circle A193 centre (673.1, 31.115) radius 2.0828 projected
  circle A194 centre (673.1, 56.515) radius 2.0828 projected
  circle A195 centre (673.1, 81.915) radius 2.0828 projected
  circle A196 centre (673.1, 107.315) radius 2.0828 projected
  circle A197 centre (673.1, 132.715) radius 2.0828 projected
  circle A198 centre (673.1, 158.115) radius 2.0828 projected
  circle A199 centre (673.1, 183.515) radius 2.0828 projected
  circle A200 centre (673.1, 208.915) radius 2.0828 projected
  circle A201 centre (673.1, 234.315) radius 2.0828 projected
  circle A202 centre (673.1, 259.715) radius 2.0828 projected
  circle A203 centre (673.1, 285.115) radius 2.0828 projected
  circle A204 centre (673.1, 310.515) radius 2.0828 projected
  circle A205 centre (673.1, 335.915) radius 2.0828 projected
  circle A206 centre (673.1, 361.315) radius 2.0828 projected
  circle A207 centre (673.1, 386.715) radius 2.0828 projected
  circle A208 centre (673.1, 412.115) radius 2.0828 projected
  circle A209 centre (673.1, 437.515) radius 2.0828 projected
  circle A210 centre (673.1, 462.915) radius 2.0828 projected
  circle A211 centre (673.1, 488.315) radius 2.0828 projected
  line L128 (0, 0) -> (685.8, 0) projected
  line L129 (685.8, 0) -> (685.8, 516.255) projected
  line L130 (685.8, 516.255) -> (0, 516.255) projected
  line L131 (0, 516.255) -> (0, 0) projected
equation "\"d17\" = Thickness"
equation "\"d29\" = Thickness"
equation "\"d65\" = Thickness"
equation "\"d60\" = BendRadius"
equation "\"d61\" = BendReliefWidth"
equation "\"d63\" = MinimumRemnant"
equation "\"d62\" = BendReliefDepth"
equation "\"d64\" = BendRadius"
equation "\"BendRadius\" = Thickness"
equation "\"BendReliefWidth\" = Thickness"
equation "\"BendReliefDepth\" = 0.5 * Thickness"
equation "\"CornerReliefSize\" = 4 * Thickness"
equation "\"MinimumRemnant\" = 2 * Thickness"
equation "\"TransitionRadius\" = BendRadius"
equation "\"JacobiRadiusSize\" = Thickness"
equation "\"GapSize\" = Thickness"
equation "\"d2\" = BendRadius"
equation "\"Thickness\" = 1.5875"
body "Solid1"
